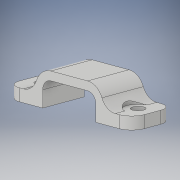
# Autodesk Inventor part: large-cable-clip
Saved by Autodesk Inventor 2018 (Build 220112000, 112)
## iProperties
Created: 2020-01-09
Part Number: large-cable-clip
Material: Generic
Document SubType Name: Modeling
Designer: Vinnie Caprarola
Density: 1 g/cm^3
Appearance: Default
Author: Vinnie Caprarola
Autodesk Inventor part; units mm, degrees
ref_plane "YZ Plane" through (0, 0, 0) normal (1, 0, 0) x (0, 1, 0)
ref_plane "XZ Plane" through (0, 0, 0) normal (0, 1, 0) x (-1, 0, 0)
ref_plane "XY Plane" through (0, 0, 0) normal (0, 0, 1) x (1, 0, 0)
sketch "Sketch1" plane through (0, 0, 0) normal (0, 0, 1) x (1, 0, 0)
  line L0 (0, 0) -> (26, 0)
  line L1 (26, 0) -> (26, 3)
  line L2 (22, 7) -> (4, 7)
  line L3 (0, 3) -> (0, 0)
  arc A0 (4, 7) -> (0, 3) centre (4, 3) ccw
  arc A1 (26, 3) -> (22, 7) centre (22, 3) ccw
  line L4 (4, 10.5) -> (22, 10.5)
  arc A2 (29.5, 3) -> (22, 10.5) centre (22, 3) ccw
  line L5 (29.5, 3) -> (29.5, -3.5)
  line L6 (29.5, -3.5) -> (-3.5, -3.5)
  line L7 (-3.5, -3.5) -> (-3.5, 3)
  arc A3 (4, 10.5) -> (-3.5, 3) centre (4, 3) ccw
  line L8 (0, 0) -> (0, -3.5)
  line L9 (26, 0) -> (26, -3.5)
  line L10 (-3.5, -3.5) -> (-17.5, -3.5)
  line L11 (-17.5, -3.5) -> (-17.5, 1.5)
  line L12 (-17.5, 1.5) -> (-3.5, 1.5)
  line L13 (-3.5, 1.5) -> (-3.5, -3.5)
  line L14 (29.5, -3.5) -> (43.5, -3.5)
  line L15 (43.5, -3.5) -> (43.5, 1.5)
  line L16 (43.5, 1.5) -> (29.5, 1.5)
  line L17 (29.5, 1.5) -> (29.5, -3.5)
  point P0 (26, 7)
  point P1 (0, 7)
  dimension "d0" = 26
  dimension "d1" = 7
  dimension "d2" = 4
  dimension "d3" = 3.5
  dimension "d6" = 14
  dimension "d7" = 5
  dimension "d8" = 14
  dimension "d9" = 5
  constraints: 36 end point, 9 parallel, 8 point on circle, 6 point on line, 5 perpendicular, 4 centre point, 4 tangent, 3 horizontal, 1 equal radius, 5 other
  measures "d0" distance of point (0, 7) point (26, 7)
  measures "d1" distance of point (26, 7) L0.end
  measures "d2" radius of A0
  measures "d3" distance between parallel lines of L2 L4
  measures "d6" distance of L11.end L12.end
  measures "d7" distance of L10.end L11.end
  measures "d8" distance of L16.end L15.end
  measures "d9" distance of L15.end L14.end
extrude "Extrusion2" add sketch "Sketch1" along normal blind 20 contours L8 L6 L7 A3 L4 A2 L5 L9 L1 A1 L2 A0 L3 | L10 L11 L12 L7 | L5 L16 L15 L14
fillet "Fillet1" radius 7 2 edges at (29.5, 1.5, 10) (-3.5, 1.5, 10)
fillet "Fillet3" radius 6 4 edges at (-17.5, -1, 20) (-17.5, -1, 0) (43.5, -1, 20) (43.5, -1, 0)
sketch "Sketch2" plane through (35.4164, 1.5, 20) normal (0, 1, 0) x (1, 0, 0)
  circle A0 centre (1.0836, 10) radius 2.75
  line L0 (8.0836, 14) -> (8.0836, 6) projected
  circle A1 centre (1.0836, 10) radius 5.5
  line L1 (-13.4164, 20) -> (-31.4164, 20) projected
  line L2 (-22.4164, 20) -> (-22.4164, 23.3018)
  circle A2 centre (-45.9164, 10) radius 2.75
  circle A3 centre (-45.9164, 10) radius 5.5
  point P0 (-35.4164, 20)
  point P1 (8.0836, 10)
  dimension "d16" = 7
  dimension "d17" = 5.5
  dimension "d18" = 11
  constraints: 4 centre point, 2 coincident, 2 end point, 2 midpoint, 2 symmetric about line, 1 horizontal alignment, 1 vertical, 2 other
  measures "d16" distance from line of A0.centre L0
  measures "d17" diameter of A0
  measures "d18" diameter of A1
extrude "Extrusion3" cut sketch "Sketch2" against normal through all contours A0 | A2
extrude "Extrusion4" cut sketch "Sketch2" along normal through all contours A0 | A1 | A2 | A3
body "Solid2"
